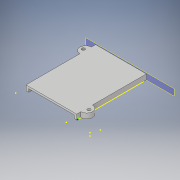
# Autodesk Inventor part: Unterteil_fertig2
Saved by Autodesk Inventor 2017 (Build 210142000, 142)
## iProperties
Part Number: Unterteil_fertig2
Material: Generisch
Document SubType Name: Modeling
Designer: Fynn
Density: 1 g/cm^3
Appearance: Vorgabe
Author: Fynn
Autodesk Inventor part; units mm, degrees
ref_plane "YZ Plane" through (0, 0, 0) normal (1, 0, 0) x (0, 1, 0)
ref_plane "XZ Plane" through (0, 0, 0) normal (0, 1, 0) x (-1, 0, 0)
ref_plane "XY Plane" through (0, 0, 0) normal (0, 0, 1) x (1, 0, 0)
sketch "Skizze1" plane through (0, 0, 0) normal (0, 0, 1) x (1, 0, 0)
  line L0 (-34.2467, 13.3525) -> (-93.0967, 13.3525)
  line L1 (-93.0967, 13.3525) -> (-93.0967, 100.3525)
  line L2 (-93.0967, 100.3525) -> (-34.2467, 100.3525)
  line L3 (-34.2467, 100.3525) -> (-34.2467, 13.3525)
  point P0 (0, 0)
  dimension "d0" = 58.85
  dimension "d1" = 87
  constraints: 8 end point, 2 parallel, 1 horizontal, 1 perpendicular
  measures "d0" distance of L0.start L0.end
  measures "d1" distance of L2.end L0.start
extrude "Extrusion1" add sketch "Skizze1" along normal blind 3.5
sketch "Skizze2" plane through (0, 0, 3.5) normal (0, 0, 1) x (1, 0, 0)
  line L0 (-93.0967, 13.3525) -> (-34.2467, 13.3525) projected
  line L1 (-93.0967, 13.3525) -> (-96.5967, 13.3525)
  line L2 (-96.5967, 13.3525) -> (-96.5967, 103.8525)
  line L3 (-96.5967, 103.8525) -> (-30.7467, 103.8525)
  line L4 (-34.2467, 100.3525) -> (-93.0967, 100.3525) projected
  line L5 (-30.7467, 103.8525) -> (-30.7467, 13.3525)
  line L6 (-30.7467, 13.3525) -> (-34.2467, 13.3525)
  line L7 (-34.2467, 13.3525) -> (-34.2467, 100.3525) projected
  line L8 (-34.2467, 13.3525) -> (-34.2467, 100.3525)
  line L9 (-34.2467, 100.3525) -> (-93.0967, 100.3525)
  line L10 (-93.0967, 100.3525) -> (-93.0967, 13.3525)
  line L11 (-30.7467, 13.3525) -> (-30.7467, 9.8525)
  line L12 (-30.7467, 9.8525) -> (-96.5967, 9.8525)
  line L13 (-96.5967, 9.8525) -> (-96.5967, 13.3525)
  line L14 (-30.7467, 13.3525) -> (-96.5967, 13.3525)
  point P0 (0, 0)
  dimension "d4" = 3.5
  dimension "d5" = 3.5
  dimension "d6" = 3.5
  dimension "d7" = 3.5
  constraints: 24 end point, 7 perpendicular, 4 point on line, 1 collinear, 1 horizontal, 1 parallel
  measures "d4" distance of L0.start L1.end
  measures "d5" distance between parallel lines of L4 L3
  measures "d6" distance between parallel lines of L5 L7
  measures "d7" distance between parallel lines of L12 L0
extrude "Extrusion2" add sketch "Skizze2" against normal blind 5.6 contours L0 L6 L11 L12 L13 L1
sketch "Skizze3" plane through (0, 0, 0) normal (0, 0, -1) x (-1, 0, 0)
  line L0 (30.7467, 15.473) -> (30.7467, 103.8525)
  line L1 (30.7467, 103.8525) -> (96.5967, 103.8525)
  line L2 (34.2467, 100.3525) -> (93.0967, 100.3525) projected
  line L3 (96.5967, 103.8525) -> (96.5967, 13.3525)
  line L4 (93.0967, 100.3525) -> (93.0967, 13.3525) projected
  line L5 (34.2467, 100.3525) -> (34.2467, 13.3525) projected
  line L6 (30.7467, 13.3525) -> (30.7467, 15.473)
  line L7 (30.7467, 13.3525) -> (34.2467, 13.3525) projected
  line L8 (30.7467, 13.3525) -> (34.2467, 13.3525)
  line L9 (34.2467, 13.3525) -> (34.2467, 100.3525) projected
  line L10 (34.2467, 13.3525) -> (34.2467, 100.3525)
  line L11 (34.2467, 100.3525) -> (93.0967, 100.3525)
  line L12 (34.2467, 13.3525) -> (93.0967, 13.3525) projected
  line L13 (93.0967, 13.3525) -> (96.5967, 13.3525) projected
  line L14 (93.0967, 13.3525) -> (96.5967, 13.3525)
  line L15 (96.5967, 13.3525) -> (96.5967, 103.8525)
  point P0 (0, 0)
  dimension "d10" = 3.5
  dimension "d11" = 3.5
  dimension "d12" = 3.5
  constraints: 18 end point, 4 parallel, 3 collinear, 1 horizontal, 1 vertical
  measures "d10" distance between parallel lines of L3 L4
  measures "d11" distance between parallel lines of L1 L2
  measures "d12" distance between parallel lines of L5 L0
extrude "Extrusion3" add sketch "Skizze3" along normal blind 4.1 contours L0 L1 L3 L13 L4 L2 L5 L7 L6
sketch "Skizze4" plane through (0, 0, 0) normal (0, 0, 1) x (1, 0, 0)
  line L0 (-34.2467, 13.3525) -> (-93.0967, 13.3525) projected
  line L1 (-96.5967, 9.8525) -> (-96.5967, 13.3525) projected
  line L2 (-93.0967, 13.3525) -> (-96.5967, 13.3525)
  line L3 (-96.5967, 103.8525) -> (-30.7467, 103.8525) projected
  line L4 (-96.5967, 13.3525) -> (-96.5967, 103.8525)
  line L5 (-96.5967, 103.8525) -> (-30.7467, 103.8525)
  line L6 (-30.7467, 103.8525) -> (-30.7467, 13.3525) projected
  line L7 (-30.7467, 103.8525) -> (-30.7467, 13.3525)
  line L8 (-34.2467, 100.3525) -> (-34.2467, 13.3525) projected
  line L9 (-30.7467, 13.3525) -> (-34.2467, 13.3525)
  line L10 (-34.2467, 100.3525) -> (-93.0967, 100.3525) projected
  line L11 (-34.2467, 13.3525) -> (-34.2467, 100.3525)
  line L12 (-34.2467, 100.3525) -> (-93.0967, 100.3525)
  line L13 (-93.0967, 100.3525) -> (-93.0967, 13.3525)
  point P0 (0, 0)
  constraints: 16 end point, 4 perpendicular, 3 collinear, 1 horizontal
extrude "Extrusion4" add sketch "Skizze4" along normal blind 3.5 contours L8 L10 L13 L2 L4 L3 L6 L9
sketch "Skizze5" plane through (-96.5967, 103.8525, -4.1) normal (0, 1, 0) x (1, 0, 0)
  line L0 (62.35, 0) -> (3.5, 0) projected
  line L1 (24.85, 0) -> (41.85, 0)
  line L2 (41.85, 0) -> (41.85, -2)
  line L3 (41.85, -2) -> (24.85, -2)
  line L4 (24.85, -2) -> (24.85, 0)
  line L5 (65.85, -7.6) -> (65.85, 0) projected
  line L6 (0, -7.6) -> (0, 0) projected
  point P0 (96.5967, -4.1)
  dimension "d17" = 17
  dimension "d18" = 24
  dimension "d19" = 2
  dimension "d40" = 24.85
  constraints: 8 end point, 2 parallel, 1 horizontal, 1 perpendicular, 1 point on line
  measures "d17" distance of L2.end L3.end
  measures "d18" distance between parallel lines of L5 L2
  measures "d19" distance of L1.end L2.end
  measures "d40" distance between parallel lines of L4 L6
extrude "Extrusion5" cut sketch "Skizze5" against normal blind 3.5
sketch "Skizze7" plane through (0, 0, -4.1) normal (0, 0, -1) x (-1, 0, 0)
  line L0 (30.7467, 9.8525) -> (30.7467, 103.8525) projected
  line L1 (30.7467, 9.8525) -> (96.5967, 9.8525) projected
  line L2 (96.5967, 13.3525) -> (96.5967, 103.8525) projected
  arc A0 (96.5967, 83.3525) -> (96.5967, 98.3525) centre (96.5967, 90.8525) ccw
  line L3 (96.5967, 103.8525) -> (71.7467, 103.8525) projected
  point P0 (0, 0)
  point P1 (30.7467, 15.3525)
  point P2 (30.7467, 30.3525)
  dimension "d24" = 15
  dimension "d25" = 13
  constraints: 5 point on line, 2 point on circle, 1 centre point
  measures "d24" diameter of A0
  measures "d25" distance from line of L3 A0.centre
sketch "Skizze8" plane through (-30.7467, 9.8525, 3.5) normal (1, 0, 0) x (0, 0, -1)
  point P0 (3.5, -9.8525)
extrude "Extrusion6" [suppressed]
sketch "Skizze9" plane through (0, 0, -4.1) normal (0, 0, -1) x (-1, 0, 0)
  circle A0 centre (27.7467, 22.8525) radius 2
  line L0 (30.7467, 103.8525) -> (30.7467, 13.3525) projected
  point P0 (0, 0)
  point P1 (30.7467, 22.8525)
  point P2 (30.7467, 15.3525)
  dimension "d28" = 7.5
  dimension "d29" = 4
  dimension "d30" = 3
  constraints: 1 centre point
  measures "d28" distance of point (30.747, 22.853) point (30.747, 15.353)
  measures "d29" diameter of A0
  measures "d30" distance from line of L0 A0.centre
extrude "Extrusion7" cut sketch "Skizze9" against normal through all
sketch "Skizze10" plane through (0, 0, -4.1) normal (0, 0, -1) x (-1, 0, 0)
  circle A0 centre (99.5967, 90.8525) radius 2
  line L0 (96.5967, 13.3525) -> (96.5967, 103.8525) projected
  point P0 (0, 0)
  point P1 (96.5967, 98.3525)
  dimension "d33" = 4
  dimension "d34" = 3
  constraints: 1 centre point
  measures "d33" diameter of A0
  measures "d34" distance from line of L0 A0.centre
extrude "Extrusion8" cut sketch "Skizze10" against normal through all
sketch "Skizze11" plane through (0, 0, 3.5) normal (0, 0, 1) x (1, 0, 0)
  point P0 (0, 0)
sketch "Skizze12" plane through (-30.7467, 9.8525, 3.5) normal (1, 0, 0) x (0, 0, -1)
  line L0 (7.6, 3.5) -> (7.6, 94) projected
  line L1 (7.6, 3.5) -> (0, 3.5)
  line L2 (0, 3.5) -> (0, 0)
  line L3 (0, 0) -> (7.6, 0)
  line L4 (7.6, 0) -> (7.6, 3.5)
  point P0 (3.5, -9.8525)
  constraints: 8 end point, 2 parallel, 1 horizontal, 1 perpendicular
extrude "Extrusion9" cut sketch "Skizze12" against normal through all
sketch "Skizze13" plane through (-30.7467, 13.3525, 3.5) normal (1, 0, 0) x (0, 0, -1)
  line L0 (7.6, 87) -> (7.6, 0) projected
  line L1 (7.6, 0) -> (5.1687, 0)
  line L2 (5.1687, 0) -> (5.1687, 2.037)
  line L3 (5.1687, 2.037) -> (7.6, 2.037)
  line L4 (7.6, 2.037) -> (7.6, 0)
  point P0 (3.5, -13.3525)
  constraints: 8 end point, 2 parallel, 1 horizontal, 1 perpendicular
sketch "Skizze14" plane through (0, 0, 3.5) normal (0, 0, 1) x (1, 0, 0)
  line L0 (-30.7467, 103.8525) -> (-30.7467, 13.3525) projected
  arc A0 (-30.7467, 18.8525) -> (-30.7467, 33.8525) centre (-30.7467, 26.3525) ccw
  line L1 (-96.5967, 103.8525) -> (-96.5967, 13.3525) projected
  arc A1 (-96.5967, 98.3525) -> (-96.5967, 83.3525) centre (-96.5967, 90.8525) ccw
  line L2 (-96.5967, 13.3525) -> (-30.7467, 13.3525) projected
  circle A2 centre (-27.7467, 26.3525) radius 2
  circle A3 centre (-99.5967, 90.8525) radius 2
  point P0 (0, 0)
  dimension "d41" = 15
  dimension "d42" = 15
  dimension "d43" = 13
  dimension "d44" = 13
  dimension "d45" = 3
  dimension "d46" = 4
  dimension "d47" = 3
  dimension "d48" = 4
  constraints: 6 point on line, 4 centre point, 4 point on circle, 2 coincident
  measures "d41" diameter of A0
  measures "d42" diameter of A1
  measures "d43" distance of L1.start A1.centre
  measures "d44" distance from line of L2 A0.centre
  measures "d45" distance of A0.centre point (-27.747, 26.353)
  measures "d46" diameter of A2
  measures "d47" distance from line of point (-99.597, 90.853) L1
  measures "d48" diameter of A3
sketch "Skizze15" plane through (-96.5967, 13.3525, 3.5) normal (-1, 0, 0) x (0, 0, 1)
  point P0 (-3.5, -13.3525)
extrude "Extrusion10" add sketch "Skizze14" against normal blind 7.6
sketch "Skizze16" plane through (-93.0967, 13.3525, 0) normal (0, -1, 0) x (1, 0, 0)
  point P0 (93.0967, 0)
sketch "Skizze17" plane through (0, 0, 3.5) normal (0, 0, 1) x (1, 0, 0)
  line L0 (-13.2494, 3.641) -> (-122.0727, 3.641)
  line L1 (-122.0727, 3.641) -> (-122.0727, 119.9278)
  line L2 (-122.0727, 119.9278) -> (-13.2494, 119.9278)
  line L3 (-13.2494, 119.9278) -> (-13.2494, 3.641)
  point P0 (0, 0)
  constraints: 8 end point, 2 parallel, 1 horizontal, 1 perpendicular
extrude "Extrusion11" cut sketch "Skizze17" against normal blind 1
sketch "Skizze18" plane through (0, 0, 0) normal (0, 0, -1) x (-1, 0, 0)
  point P0 (0, 0)
ref_plane "Arbeitsebene1" through (-96.5967, 103.8525, -4.1) normal (0, 1, 0) x (1, 0, 0)
sketch "Skizze19" plane through (-96.5967, 103.8525, -4.1) normal (0, 1, 0) x (1, 0, 0)
  line L0 (0, -6.6) -> (0, 0) projected
  line L1 (0, 0) -> (24.85, 0) projected
  line L2 (0, -6.6) -> (65.85, -6.6) projected
  line L3 (65.85, -6.6) -> (65.85, 0) projected
  line L4 (41.85, 0) -> (65.85, 0) projected
  line L5 (24, -2) -> (41.85, -2)
  line L6 (41.85, -2) -> (41.85, 5.2977)
  line L7 (41.85, 5.2977) -> (24, 5.2977)
  line L8 (24, 5.2977) -> (24, -2)
  point P0 (96.5967, -4.1)
  dimension "d54" = 24
  dimension "d55" = 24
  dimension "d56" = 2
  constraints: 8 end point, 2 parallel, 1 horizontal, 1 perpendicular
  measures "d54" distance between parallel lines of L0 L8
  measures "d55" distance between parallel lines of L3 L6
  measures "d56" distance between parallel lines of L1 L5
extrude "Extrusion12" cut sketch "Skizze19" against normal blind 10 contours L8 L7 L6 L5
